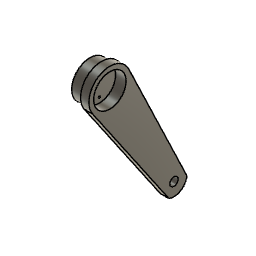
thigh_right v2 v0 v1 (Autodesk Fusion 360 design; units mm, degrees)
Autodesk Fusion 360 part; units mm, degrees
note: some values were not read from the file. Set by a fixed rule: which sketch regions a step uses.
sketch "Sketch1" plane through (0, 0, 0) normal (1, 0, 0) x (0, 1, 0)
  circle A0 centre (0, 0) radius 20
  line L0 (0, 0) -> (65, -112.5833)
  line L1 (0, 0) -> (130, 0) construction
  line L2 (-16.4974, -11.3065) -> (56.3397, -117.5833)
  line L3 (56.3397, -117.5833) -> (65, -112.5833)
  line L4 (65, -112.5833) -> (73.6603, -107.5833)
  line L5 (73.6603, -107.5833) -> (18.0404, 8.6339)
  circle A1 centre (0, 0) radius 17.5
  circle A2 centre (61.25, -106.0881) radius 12.5
  circle A3 centre (61.25, -106.0881) radius 7.5
  dimension "d1" = 40
  dimension "d2" = 60
  dimension "d3" = 130
  dimension "d4" = 10
  dimension "d5" = 10
  dimension "d6" = 35
  dimension "d7" = 25
  dimension "d8" = 15
  constraint coincident A0.centre L0.start
  constraint horizontal L1
  constraint coincident A0 L2.start
  constraint perpendicular L0 L4
  constraint coincident A0 L5.end
  constraint tangent A0 L5
  constraint tangent A0 L2
  constraint perpendicular L0 L3
  constraint concentric A0 A1
  constraint coincident L2.end A2
  constraint coincident L4.end A2
  constraint concentric A2 A3
  measures "d1" diameter of A0
  measures "d2" angle of L0 L1
  measures "d3" distance of A0.centre L0.end
  measures "d4" distance of L0.end L2.end
  measures "d5" distance of L0.end L4.end
  measures "d6" diameter of A1
  measures "d7" diameter of A2
  measures "d8" diameter of A3
extrude "Extrude1" add sketch "Sketch1" along normal mid plane 8 contours A0 | A0 L0 L5 A2 | A0 L0 L2 A2 | L0 L4 L5 A2 A3 | L0 L2 L3 A2 A3 | L3 L4 A2 | L0 A3 | L0 A3 | A1
extrude "Extrude2" add sketch "Sketch1" against normal blind 15 contours A1
extrude "Extrude3" add sketch "Sketch1" along normal mid plane 20 contours L0 A3 | L0 A3
extrude "Extrude4" cut 1 faces at (10, 60.7061, -108.3596) along direction (-1, 0, 0) blind 6
extrude "Extrude5" cut 1 faces at (-10, 60.6937, -103.8711) along direction (1, 0, 0) blind 6
sketch "Sketch2" plane through (-15, 0, 0) normal (-1, 0, 0) x (0, -1, 0)
  circle A0 centre (0, 0) radius 17.5
  line L0 (0, 0) -> (0, 10.5)
  line L1 (0, 0) -> (0, -10.5)
  circle A1 centre (0, 10.5) radius 1
  circle A2 centre (0, -10.5) radius 1
  dimension "d19" = 10.5
  dimension "d20" = 10.5
  dimension "d21" = 2
  dimension "d22" = 2
  constraint coincident A0.centre L0.start
  constraint vertical L0
  constraint parallel L0 L1
  constraint coincident L0.end A1.centre
  constraint coincident L1.end A2.centre
  measures "d19" distance of A0.centre L0.end
  measures "d20" distance of A0.centre L1.end
  measures "d21" diameter of A1
  measures "d22" diameter of A2
extrude "Extrude6" cut sketch "Sketch2" against normal blind 26 contours A1 | A2
sketch "Sketch3" plane through (-15, 0, 0) normal (-1, 0, 0) x (0, -1, 0)
  circle A0 centre (0, 10.5) radius 1
  circle A1 centre (0, -10.5) radius 1
  circle A2 centre (0, 0) radius 17.5
  circle A3 centre (0, 0) radius 15.5
  dimension "d25" = 31
  constraint coincident A2.centre A3.centre
  measures "d25" diameter of A3
extrude "Extrude7" cut sketch "Sketch3" against normal blind 2 contours A3
sketch "Sketch4" plane through (4, 0, 0) normal (1, 0, 0) x (0, 1, 0)
  circle A0 centre (0, 10.5) radius 1
  circle A1 centre (0, -10.5) radius 1
  line L0 (73.6603, -107.5833) -> (18.0404, 8.6339)
  arc A2 (18.0404, 8.6339) -> (-16.4974, -11.3065) centre (0, 0) ccw
  line L1 (-16.4974, -11.3065) -> (56.3397, -117.5833)
  arc A3 (56.3397, -117.5833) -> (73.6603, -107.5833) centre (61.25, -106.0881) ccw
  circle A4 centre (0, 0) radius 15.5
  circle A5 centre (0, 0) radius 15.5
  constraint concentric A2 A5
extrude "Extrude8" cut sketch "Sketch4" against normal blind 10 contours A4 A5
sketch "Sketch5" plane through (4, 0, 0) normal (1, 0, 0) x (0, 1, 0)
  circle A0 centre (0, 0) radius 15.5
  line L0 (73.6603, -107.5833) -> (18.0404, 8.6339)
  arc A1 (18.0404, 8.6339) -> (-16.4974, -11.3065) centre (0, 0) ccw
  line L1 (-16.4974, -11.3065) -> (56.3397, -117.5833)
  arc A2 (56.3397, -117.5833) -> (73.6603, -107.5833) centre (61.25, -106.0881) ccw
  circle A3 centre (61.25, -106.0881) radius 12.5
  circle A4 centre (61.25, -106.0881) radius 4
  dimension "d30" = 8
  constraint concentric A3 A4
  measures "d30" diameter of A4
extrude "Extrude9" cut sketch "Sketch5" against normal blind 10 contours A4
equation "d19 = ( 21 / 2 ) * 1 mm"
